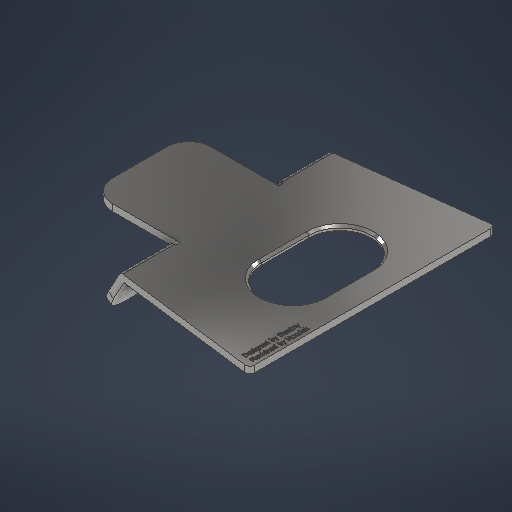
# Autodesk Inventor part: MK_5_rust_helma1
Saved by Autodesk Inventor 2025.3 (Build 293356000, 356)
## iProperties
Created: 2025-04-03
Part Number: MK_5_rust_helma1
Material: Ocel
Document SubType Name: Modeling
Designer: kolom_rupe2o
Density: 7.85 g/cm^3
Appearance: Ocel – leštěná
Author: kolom_rupe2o
Autodesk Inventor part; units mm, degrees
(part 1 of 2)
ref_plane "YZ Plane" through (0, 0, 0) normal (1, 0, 0) x (0, 1, 0)
ref_plane "XZ Plane" through (0, 0, 0) normal (0, 1, 0) x (-1, 0, 0)
ref_plane "XY Plane" through (0, 0, 0) normal (0, 0, 1) x (1, 0, 0)
sketch "Náčrt1" plane through (0, 0, 0) normal (0, 1, 0) x (-1, 0, 0)
  line L0 (0, 0) -> (0, -55)
  line L1 (0, -55) -> (32, -51)
  line L2 (32, -51) -> (32, -4)
  line L3 (32, -4) -> (0, 0)
  line L4 (12.5, -22.25) -> (12.5, -32.75) construction
  line L5 (5.5, -22.25) -> (5.5, -32.75)
  line L6 (19.5, -32.75) -> (19.5, -22.25)
  arc A0 (19.5, -22.25) -> (5.5, -22.25) centre (12.5, -22.25) ccw
  arc A1 (5.5, -32.75) -> (19.5, -32.75) centre (12.5, -32.75) ccw
  line L7 (32, -16.5) -> (52, -16.5)
  line L8 (52, -16.5) -> (52, -38.5)
  line L9 (52, -38.5) -> (32, -38.5)
  line L10 (32, -38.5) -> (32, -16.5)
  point P0 (32, -27.5)
  point P1 (0, -27.5)
  point P2 (12.5, -27.5)
  point P3 (52, -27.5)
  dimension "d0" = 47
  dimension "d1" = 55
  dimension "d2" = 32
  dimension "d3" = 12.5
  dimension "d4" = 7
  dimension "d5" = 10.5
  dimension "d6" = 22
  dimension "d7" = 20
  constraints: 24 end point, 4 midpoint, 4 parallel, 4 point on circle, 4 tangent, 3 horizontal alignment, 2 centre point, 2 vertical, 1 equal length, 1 horizontal, 1 perpendicular, 1 point on line
  measures "d0" distance of L1.end L2.end
  measures "d1" distance of L0.start L0.end
  measures "d2" distance between parallel lines of L0 L2
  measures "d3" distance between parallel lines of L2 L6
  measures "d4" radius of A1
  measures "d5" distance of L4.start L4.end
  measures "d6" distance of L7.end L8.end
  measures "d7" distance of L8.end L9.end
extrude "Vysunutí1" add sketch "Náčrt1" along normal blind 1.5
ref_plane "Pracovní rovina1" through (-52, 0, -27.5) normal (0, 0, 1) x (1, 0, 0)
ref_plane "Pracovní rovina2" through (-52, 0, -15.5) normal (0, 0, 1) x (1, 0, 0)
sketch "Náčrt3" plane through (-52, 0, -15.5) normal (0, 0, 1) x (1, 0, 0)
  line L0 (20, 0) -> (52, 0)
  line L1 (52, 0) -> (52, 1.5)
  line L2 (20, 1.5) -> (52, 1.5)
  line L3 (20, 0) -> (20, 1.5)
  line L4 (20, 0) -> (15, -8.6603)
  line L5 (15, -8.6603) -> (13.701, -7.9103)
  line L6 (13.701, -7.9103) -> (19.134, 1.5)
  line L7 (19.134, 1.5) -> (20, 1.5)
  line L8 (20, 0) -> (20, 1.5)
  line L9 (20, 0) -> (20, 1.5)
  dimension "d14" = 120
  dimension "d15" = 1.5
  dimension "d16" = 10
  constraints: 8 end point, 2 perpendicular, 1 collinear
  measures "d14" angle of L0 L4
  measures "d15" distance of L4.end L5.end
  measures "d16" distance of L0.start L4.end
extrude "Vysunutí2" add sketch "Náčrt3" along normal up to surface contours L4 L5 L6 L7 L3 surface through (-32, 0, -4) normal (-0.1240347, 0, 0.9922779)
sketch "Náčrt4" plane through (-32.866, 1.5, -15.5) normal (-0.8660254, 0.5, 0) x (0, 0, 1)
  line L0 (10.7126, -10.866) -> (11.3917, 0)
  line L1 (0, 0) -> (11.3917, 0)
  line L2 (0, 0) -> (0, -10.866)
  line L3 (0, -10.866) -> (10.7126, -10.866)
  point P0 (15.5, 15.134)
  point P1 (5.3563, -5.433)
  point P2 (0, -5.433)
  point P3 (5.3563, -10.866)
  constraints: 2 midpoint, 1 horizontal alignment, 1 vertical alignment
hole "Díra1" at (-35.5825, -3.2051, -10.1437) direction (0.8660254, -0.5, 0) diameter 3 end through all
mirror "Zrcadlit1" about plane through (-52, 0, -27.5) normal (0, 0, 1) of "Díra1", "Vysunutí2"
fillet "Zaoblení1" radius 1 2 edges at (-32.866, 1.5, -45.1959) (-32.866, 1.5, -9.8041)
fillet "Zaoblení2" radius 5 6 edges at (-37.6495, -8.2853, -4.7062) (-37.6495, -8.2853, -15.5) (-37.6495, -8.2853, -39.5) (-37.6495, -8.2853, -50.2938) (-52, 0.75, -16.5) (-52, 0.75, -38.5)
fillet "Zaoblení3" radius 1 2 edges at (0, 0.75, -55) (0, 0.75, 0)
chamfer "Zkosení1" distance 0.5 angle 45 8 edges at (-19.5, 1.5, -27.5) (-12.5, 1.5, -39.75) (-5.5, 1.5, -27.5) (-12.5, 1.5, -15.25) (-19.5, 0, -27.5) (-12.5, 0, -39.75) (-5.5, 0, -27.5) (-12.5, 0, -15.25)
sketch "Náčrt6" plane through (0, 1.5, 0) normal (0, 1, 0) x (1, 0, 0)
  arc A0 (-1.124, 0.1405) -> (0, 1.1328) centre (-1, 1.1328) ccw
  line L0 (0, 1.1328) -> (0, 53.8672)
  arc A1 (0, 53.8672) -> (-1.124, 54.8595) centre (-1, 53.8672) ccw
  line L1 (-1.124, 54.8595) -> (-32.2887, 50.9639)
  line L2 (-32.2887, 39.5) -> (-32.2887, 50.9639)
  line L3 (-32, 39.5) -> (-32.2887, 39.5)
  line L4 (-32, 39.5) -> (-32, 38.5)
  line L5 (-32, 38.5) -> (-47, 38.5)
  arc A2 (-47, 38.5) -> (-52, 33.5) centre (-47, 33.5) ccw
  line L6 (-52, 33.5) -> (-52, 21.5)
  arc A3 (-52, 21.5) -> (-47, 16.5) centre (-47, 21.5) ccw
  line L7 (-47, 16.5) -> (-32, 16.5)
  line L8 (-32, 16.5) -> (-32, 15.5)
  line L9 (-32, 15.5) -> (-32.2887, 15.5)
  line L10 (-32.2887, 4.0361) -> (-32.2887, 15.5)
  line L11 (-32.2887, 4.0361) -> (-1.124, 0.1405)
  line L12 (-20, 32.75) -> (-20, 22.25)
  arc A4 (-5, 32.75) -> (-20, 32.75) centre (-12.5, 32.75) ccw
  line L13 (-5, 22.25) -> (-5, 32.75)
  arc A5 (-20, 22.25) -> (-5, 22.25) centre (-12.5, 22.25) ccw
  line L14 (-3.5, 1.6328) -> (-3.5, 16.6328) construction
  line L15 (-3.5, 16.6328) -> (0, 16.6328) construction
  line L16 (0, 16.6328) -> (0, 1.6328) construction
  line L17 (0, 1.6328) -> (-3.5, 1.6328) construction
  spline S0 degree 2 poles (-2.9546, 2.5226) (-2.8177, 2.5226) (-2.5972, 2.4116) (-2.5357, 2.3184) knots 0 0 0 1 2 2 2
  spline S1 degree 2 poles (-2.5357, 2.3184) (-2.4878, 2.2422) (-2.4554, 2.0858) (-2.4554, 1.9642) knots 0 0 0 1 2 2 2
  line L18 (-2.4554, 1.9642) -> (-2.4554, 1.7341)
  line L19 (-2.4554, 1.7341) -> (-3.4554, 1.7341)
  line L20 (-3.4554, 1.7341) -> (-3.4554, 1.9618)
  spline S2 degree 2 poles (-3.4554, 1.9618) (-3.4554, 2.1028) (-3.4133, 2.2633) (-3.376, 2.32) knots 0 0 0 1 2 2 2
  spline S3 degree 2 poles (-3.376, 2.32) (-3.312, 2.4164) (-3.1005, 2.5226) (-2.9546, 2.5226) knots 0 0 0 1 2 2 2
  spline S4 degree 2 poles (-2.9562, 2.384) (-3.0713, 2.384) (-3.2342, 2.3078) (-3.2804, 2.2325) knots 0 0 0 1 2 2 2
  spline S5 degree 2 poles (-3.2804, 2.2325) (-3.312, 2.179) (-3.3404, 2.0582) (-3.3404, 1.9683) knots 0 0 0 1 2 2 2
  line L21 (-3.3404, 1.9683) -> (-3.3404, 1.867)
  line L22 (-3.3404, 1.867) -> (-2.5705, 1.867)
  line L23 (-2.5705, 1.867) -> (-2.5705, 1.9683)
  spline S6 degree 2 poles (-2.5705, 1.9683) (-2.5705, 2.0566) (-2.5989, 2.1903) (-2.637, 2.2446) knots 0 0 0 1 2 2 2
  spline S7 degree 2 poles (-2.637, 2.2446) (-2.684, 2.3143) (-2.8395, 2.384) (-2.9562, 2.384) knots 0 0 0 1 2 2 2
  spline S8 degree 2 poles (-2.4384, 2.9829) (-2.4384, 2.803) (-2.6402, 2.6052) (-2.8266, 2.6052) knots 0 0 0 1 2 2 2
  spline S9 degree 2 poles (-2.8266, 2.6052) (-3.0097, 2.6052) (-3.2269, 2.7973) (-3.2269, 2.9521) knots 0 0 0 1 2 2 2
  spline S10 degree 2 poles (-3.2269, 2.9521) (-3.2269, 3.0218) (-3.1864, 3.1295) (-3.1434, 3.1692) knots 0 0 0 1 2 2 2
  spline S11 degree 2 poles (-3.1434, 3.1692) (-3.1005, 3.2098) (-2.9765, 3.2527) (-2.8865, 3.2527) knots 0 0 0 1 2 2 2
  line L24 (-2.8865, 3.2527) -> (-2.8177, 3.2527)
  line L25 (-2.8177, 3.2527) -> (-2.8177, 2.7333)
  spline S12 degree 2 poles (-2.8177, 2.7333) (-2.6872, 2.7333) (-2.5486, 2.8645) (-2.5486, 2.9812) knots 0 0 0 1 2 2 2
  spline S13 degree 2 poles (-2.5486, 2.9812) (-2.5486, 3.0226) (-2.5673, 3.1028) (-2.5818, 3.1352) knots 0 0 0 1 2 2 2
  spline S14 degree 2 poles (-2.5818, 3.1352) (-2.5981, 3.1692) (-2.6264, 3.2163) (-2.6394, 3.2316) knots 0 0 0 1 2 2 2
  line L26 (-2.6394, 3.2316) -> (-2.6394, 3.2389)
  line L27 (-2.6394, 3.2389) -> (-2.5016, 3.2389)
  spline S15 degree 2 poles (-2.5016, 3.2389) (-2.4927, 3.2171) (-2.4668, 3.1506) (-2.4595, 3.1247) knots 0 0 0 1 2 2 2
  spline S16 degree 2 poles (-2.4595, 3.1247) (-2.4489, 3.0882) (-2.4384, 3.0282) (-2.4384, 2.9829) knots 0 0 0 1 2 2 2
  spline S17 degree 2 poles (-2.9141, 3.1295) (-2.9652, 3.1279) (-3.0397, 3.1069) (-3.0648, 3.0866) knots 0 0 0 1 2 2 2
  spline S18 degree 2 poles (-3.0648, 3.0866) (-3.0932, 3.0647) (-3.1232, 2.9958) (-3.1232, 2.9448) knots 0 0 0 1 2 2 2
  spline S19 degree 2 poles (-3.1232, 2.9448) (-3.1232, 2.8945) (-3.0932, 2.824) (-3.064, 2.7949) knots 0 0 0 1 2 2 2
  spline S20 degree 2 poles (-3.064, 2.7949) (-3.034, 2.7665) (-2.9619, 2.7373) (-2.9141, 2.7333) knots 0 0 0 1 2 2 2
  line L28 (-2.9141, 2.7333) -> (-2.9141, 3.1295)
  spline S21 degree 2 poles (-2.4376, 3.5833) (-2.4376, 3.508) (-2.4781, 3.3775) (-2.5008, 3.3346) knots 0 0 0 1 2 2 2
  line L29 (-2.5008, 3.3346) -> (-2.6426, 3.3346)
  line L30 (-2.6426, 3.3346) -> (-2.6426, 3.341)
  spline S22 degree 2 poles (-2.6426, 3.341) (-2.6297, 3.3573) (-2.5989, 3.401) (-2.5818, 3.4375) knots 0 0 0 1 2 2 2
  spline S23 degree 2 poles (-2.5818, 3.4375) (-2.5665, 3.4691) (-2.5438, 3.5469) (-2.5438, 3.5882) knots 0 0 0 1 2 2 2
  spline S24 degree 2 poles (-2.5438, 3.5882) (-2.5438, 3.6182) (-2.5575, 3.6871) (-2.5689, 3.7033) knots 0 0 0 1 2 2 2
  spline S25 degree 2 poles (-2.5689, 3.7033) (-2.5843, 3.7268) (-2.6191, 3.7479) (-2.6548, 3.7479) knots 0 0 0 1 2 2 2
  spline S26 degree 2 poles (-2.6548, 3.7479) (-2.6994, 3.7479) (-2.7455, 3.6992) (-2.7609, 3.6368) knots 0 0 0 1 2 2 2
  spline S27 degree 2 poles (-2.7609, 3.6368) (-2.7666, 3.6125) (-2.7828, 3.5347) (-2.7917, 3.5015) knots 0 0 0 1 2 2 2
  spline S28 degree 2 poles (-2.7917, 3.5015) (-2.8169, 3.4156) (-2.9206, 3.3378) (-2.9943, 3.3378) knots 0 0 0 1 2 2 2
  spline S29 degree 2 poles (-2.9943, 3.3378) (-3.0964, 3.3378) (-3.2237, 3.491) (-3.2237, 3.6174) knots 0 0 0 1 2 2 2
  spline S30 degree 2 poles (-3.2237, 3.6174) (-3.2237, 3.6798) (-3.1929, 3.8062) (-3.1694, 3.8492) knots 0 0 0 1 2 2 2
  line L31 (-3.1694, 3.8492) -> (-3.034, 3.8492)
  line L32 (-3.034, 3.8492) -> (-3.034, 3.8427)
  spline S31 degree 2 poles (-3.034, 3.8427) (-3.0729, 3.794) (-3.1175, 3.6757) (-3.1175, 3.615) knots 0 0 0 1 2 2 2
  spline S32 degree 2 poles (-3.1175, 3.615) (-3.1175, 3.5526) (-3.0648, 3.4667) (-3.0122, 3.4667) knots 0 0 0 1 2 2 2
  spline S33 degree 2 poles (-3.0122, 3.4667) (-2.9643, 3.4667) (-2.9182, 3.5177) (-2.9036, 3.5744) knots 0 0 0 1 2 2 2
  spline S34 degree 2 poles (-2.9036, 3.5744) (-2.8963, 3.602) (-2.8817, 3.6717) (-2.8728, 3.7098) knots 0 0 0 1 2 2 2
  spline S35 degree 2 poles (-2.8728, 3.7098) (-2.8517, 3.7924) (-2.7553, 3.8767) (-2.6718, 3.8767) knots 0 0 0 1 2 2 2
  spline S36 degree 2 poles (-2.6718, 3.8767) (-2.6232, 3.8767) (-2.5373, 3.8386) (-2.5057, 3.8013) knots 0 0 0 1 2 2 2
  spline S37 degree 2 poles (-2.5057, 3.8013) (-2.4724, 3.7616) (-2.4376, 3.6603) (-2.4376, 3.5833) knots 0 0 0 1 2 2 2
  line L33 (-2.4554, 4.1231) -> (-2.4554, 3.9966)
  line L34 (-2.4554, 3.9966) -> (-3.2058, 3.9966)
  line L35 (-3.2058, 3.9966) -> (-3.2058, 4.1231)
  line L36 (-3.2058, 4.1231) -> (-2.4554, 4.1231)
  line L37 (-3.3306, 4.132) -> (-3.3306, 3.9885)
  line L38 (-3.3306, 3.9885) -> (-3.4619, 3.9885)
  line L39 (-3.4619, 3.9885) -> (-3.4619, 4.132)
  line L40 (-3.4619, 4.132) -> (-3.3306, 4.132)
  spline S38 degree 2 poles (-2.3355, 4.3354) (-2.3298, 4.3483) (-2.312, 4.3978) (-2.3047, 4.4294) knots 0 0 0 1 2 2 2
  spline S39 degree 2 poles (-2.3047, 4.4294) (-2.2958, 4.4642) (-2.2853, 4.5234) (-2.2853, 4.5582) knots 0 0 0 1 2 2 2
  spline S40 degree 2 poles (-2.2853, 4.5582) (-2.2853, 4.6166) (-2.316, 4.6976) (-2.3436, 4.7203) knots 0 0 0 1 2 2 2
  spline S41 degree 2 poles (-2.3436, 4.7203) (-2.3712, 4.7422) (-2.4433, 4.7592) (-2.4895, 4.7592) knots 0 0 0 1 2 2 2
  line L41 (-2.4895, 4.7592) -> (-2.5551, 4.7592)
  spline S42 degree 2 poles (-2.5551, 4.7592) (-2.5105, 4.7081) (-2.4684, 4.6101) (-2.4684, 4.5363) knots 0 0 0 1 2 2 2
  spline S43 degree 2 poles (-2.4684, 4.5363) (-2.4684, 4.4083) (-2.6588, 4.2568) (-2.8379, 4.2568) knots 0 0 0 1 2 2 2
  spline S44 degree 2 poles (-2.8379, 4.2568) (-2.9311, 4.2568) (-3.0754, 4.3094) (-3.1264, 4.3532) knots 0 0 0 1 2 2 2
  spline S45 degree 2 poles (-3.1264, 4.3532) (-3.1742, 4.3953) (-3.2269, 4.5112) (-3.2269, 4.5728) knots 0 0 0 1 2 2 2
  spline S46 degree 2 poles (-3.2269, 4.5728) (-3.2269, 4.6312) (-3.1994, 4.7163) (-3.1742, 4.7592) knots 0 0 0 1 2 2 2
  line L42 (-3.1742, 4.7592) -> (-3.2058, 4.7665)
  line L43 (-3.2058, 4.7665) -> (-3.2058, 4.8856)
  line L44 (-3.2058, 4.8856) -> (-2.5413, 4.8856)
  spline S47 degree 2 poles (-2.5413, 4.8856) (-2.3501, 4.8856) (-2.1718, 4.7195) (-2.1718, 4.5485) knots 0 0 0 1 2 2 2
  spline S48 degree 2 poles (-2.1718, 4.5485) (-2.1718, 4.4934) (-2.1896, 4.3783) (-2.2042, 4.3289) knots 0 0 0 1 2 2 2
  line L45 (-2.2042, 4.3289) -> (-2.3355, 4.3289)
  line L46 (-2.3355, 4.3289) -> (-2.3355, 4.3354)
  line L47 (-2.6588, 4.7592) -> (-3.0713, 4.7592)
  spline S49 degree 2 poles (-3.0713, 4.7592) (-3.094, 4.7122) (-3.1135, 4.6328) (-3.1135, 4.5931) knots 0 0 0 1 2 2 2
  spline S50 degree 2 poles (-3.1135, 4.5931) (-3.1135, 4.4975) (-2.9724, 4.3872) (-2.8404, 4.3872) knots 0 0 0 1 2 2 2
  spline S51 degree 2 poles (-2.8404, 4.3872) (-2.7156, 4.3872) (-2.5851, 4.4707) (-2.5851, 4.5647) knots 0 0 0 1 2 2 2
  spline S52 degree 2 poles (-2.5851, 4.5647) (-2.5851, 4.6141) (-2.624, 4.7179) (-2.6588, 4.7592) knots 0 0 0 1 2 2 2
  line L48 (-2.4554, 5.6579) -> (-2.4554, 5.5315)
  line L49 (-2.4554, 5.5315) -> (-2.8833, 5.5315)
  spline S53 degree 2 poles (-2.8833, 5.5315) (-2.9352, 5.5315) (-3.0243, 5.5218) (-3.0511, 5.5072) knots 0 0 0 1 2 2 2
  spline S54 degree 2 poles (-3.0511, 5.5072) (-3.0794, 5.4918) (-3.107, 5.4367) (-3.107, 5.3897) knots 0 0 0 1 2 2 2
  spline S55 degree 2 poles (-3.107, 5.3897) (-3.107, 5.3427) (-3.0567, 5.243) (-3.0162, 5.1952) knots 0 0 0 1 2 2 2
  line L50 (-3.0162, 5.1952) -> (-2.4554, 5.1952)
  line L51 (-2.4554, 5.1952) -> (-2.4554, 5.0688)
  line L52 (-2.4554, 5.0688) -> (-3.2058, 5.0688)
  line L53 (-3.2058, 5.0688) -> (-3.2058, 5.1952)
  line L54 (-3.2058, 5.1952) -> (-3.1224, 5.1952)
  spline S56 degree 2 poles (-3.1224, 5.1952) (-3.1734, 5.2519) (-3.2269, 5.3613) (-3.2269, 5.4229) knots 0 0 0 1 2 2 2
  spline S57 degree 2 poles (-3.2269, 5.4229) (-3.2269, 5.5331) (-3.081, 5.6579) (-2.9425, 5.6579) knots 0 0 0 1 2 2 2
  line L55 (-2.9425, 5.6579) -> (-2.4554, 5.6579)
  spline S58 degree 2 poles (-2.4384, 6.1611) (-2.4384, 5.9812) (-2.6402, 5.7835) (-2.8266, 5.7835) knots 0 0 0 1 2 2 2
  spline S59 degree 2 poles (-2.8266, 5.7835) (-3.0097, 5.7835) (-3.2269, 5.9756) (-3.2269, 6.1304) knots 0 0 0 1 2 2 2
  spline S60 degree 2 poles (-3.2269, 6.1304) (-3.2269, 6.2) (-3.1864, 6.3078) (-3.1434, 6.3475) knots 0 0 0 1 2 2 2
  spline S61 degree 2 poles (-3.1434, 6.3475) (-3.1005, 6.388) (-2.9765, 6.431) (-2.8865, 6.431) knots 0 0 0 1 2 2 2
  line L56 (-2.8865, 6.431) -> (-2.8177, 6.431)
  line L57 (-2.8177, 6.431) -> (-2.8177, 5.9116)
  spline S62 degree 2 poles (-2.8177, 5.9116) (-2.6872, 5.9116) (-2.5486, 6.0428) (-2.5486, 6.1595) knots 0 0 0 1 2 2 2
  spline S63 degree 2 poles (-2.5486, 6.1595) (-2.5486, 6.2009) (-2.5673, 6.2811) (-2.5818, 6.3135) knots 0 0 0 1 2 2 2
  spline S64 degree 2 poles (-2.5818, 6.3135) (-2.5981, 6.3475) (-2.6264, 6.3945) (-2.6394, 6.4099) knots 0 0 0 1 2 2 2
  line L58 (-2.6394, 6.4099) -> (-2.6394, 6.4172)
  line L59 (-2.6394, 6.4172) -> (-2.5016, 6.4172)
  spline S65 degree 2 poles (-2.5016, 6.4172) (-2.4927, 6.3953) (-2.4668, 6.3289) (-2.4595, 6.303) knots 0 0 0 1 2 2 2
  spline S66 degree 2 poles (-2.4595, 6.303) (-2.4489, 6.2665) (-2.4384, 6.2065) (-2.4384, 6.1611) knots 0 0 0 1 2 2 2
  spline S67 degree 2 poles (-2.9141, 6.3078) (-2.9652, 6.3062) (-3.0397, 6.2851) (-3.0648, 6.2649) knots 0 0 0 1 2 2 2
  spline S68 degree 2 poles (-3.0648, 6.2649) (-3.0932, 6.243) (-3.1232, 6.1741) (-3.1232, 6.1231) knots 0 0 0 1 2 2 2
  spline S69 degree 2 poles (-3.1232, 6.1231) (-3.1232, 6.0728) (-3.0932, 6.0023) (-3.064, 5.9731) knots 0 0 0 1 2 2 2
  spline S70 degree 2 poles (-3.064, 5.9731) (-3.034, 5.9448) (-2.9619, 5.9156) (-2.9141, 5.9116) knots 0 0 0 1 2 2 2
  line L60 (-2.9141, 5.9116) -> (-2.9141, 6.3078)
  line L61 (-2.4554, 7.136) -> (-2.4554, 7.0096)
  line L62 (-2.4554, 7.0096) -> (-2.5316, 7.0096)
  spline S71 degree 2 poles (-2.5316, 7.0096) (-2.5073, 6.9804) (-2.4749, 6.9375) (-2.4611, 6.9083) knots 0 0 0 1 2 2 2
  spline S72 degree 2 poles (-2.4611, 6.9083) (-2.4481, 6.8816) (-2.4344, 6.824) (-2.4344, 6.7859) knots 0 0 0 1 2 2 2
  spline S73 degree 2 poles (-2.4344, 6.7859) (-2.4344, 6.7244) (-2.4854, 6.6206) (-2.5348, 6.5842) knots 0 0 0 1 2 2 2
  spline S74 degree 2 poles (-2.5348, 6.5842) (-2.5843, 6.5477) (-2.7301, 6.5072) (-2.825, 6.5072) knots 0 0 0 1 2 2 2
  spline S75 degree 2 poles (-2.825, 6.5072) (-2.9238, 6.5072) (-3.0681, 6.5582) (-3.1224, 6.6028) knots 0 0 0 1 2 2 2
  spline S76 degree 2 poles (-3.1224, 6.6028) (-3.171, 6.6441) (-3.2269, 6.76) (-3.2269, 6.824) knots 0 0 0 1 2 2 2
  spline S77 degree 2 poles (-3.2269, 6.824) (-3.2269, 6.8799) (-3.2018, 6.9634) (-3.1759, 7.0096) knots 0 0 0 1 2 2 2
  line L63 (-3.1759, 7.0096) -> (-3.5, 7.0096)
  line L64 (-3.5, 7.0096) -> (-3.5, 7.136)
  line L65 (-3.5, 7.136) -> (-2.4554, 7.136)
  line L66 (-2.6378, 7.0096) -> (-3.0713, 7.0096)
  spline S78 degree 2 poles (-3.0713, 7.0096) (-3.094, 6.9626) (-3.111, 6.888) (-3.111, 6.8451) knots 0 0 0 1 2 2 2
  spline S79 degree 2 poles (-3.111, 6.8451) (-3.111, 6.7479) (-2.9652, 6.6376) (-2.8274, 6.6376) knots 0 0 0 1 2 2 2
  spline S80 degree 2 poles (-2.8274, 6.6376) (-2.6945, 6.6376) (-2.5543, 6.7219) (-2.5543, 6.8151) knots 0 0 0 1 2 2 2
  spline S81 degree 2 poles (-2.5543, 6.8151) (-2.5543, 6.8645) (-2.5997, 6.965) (-2.6378, 7.0096) knots 0 0 0 1 2 2 2
  spline S82 degree 2 poles (-2.8428, 8.3775) (-2.6588, 8.3775) (-2.4344, 8.1992) (-2.4344, 8.0647) knots 0 0 0 1 2 2 2
  spline S83 degree 2 poles (-2.4344, 8.0647) (-2.4344, 8.0039) (-2.4643, 7.9172) (-2.4903, 7.8751) knots 0 0 0 1 2 2 2
  line L67 (-2.4903, 7.8751) -> (-2.4554, 7.867)
  line L68 (-2.4554, 7.867) -> (-2.4554, 7.7487)
  line L69 (-2.4554, 7.7487) -> (-3.5, 7.7487)
  line L70 (-3.5, 7.7487) -> (-3.5, 7.8751)
  line L71 (-3.5, 7.8751) -> (-3.1272, 7.8751)
  spline S84 degree 2 poles (-3.1272, 7.8751) (-3.1702, 7.9229) (-3.2269, 8.0339) (-3.2269, 8.1044) knots 0 0 0 1 2 2 2
  spline S85 degree 2 poles (-3.2269, 8.1044) (-3.2269, 8.2316) (-3.0235, 8.3775) (-2.8428, 8.3775) knots 0 0 0 1 2 2 2
  spline S86 degree 2 poles (-2.8331, 8.247) (-2.9676, 8.247) (-3.107, 8.1652) (-3.107, 8.0744) knots 0 0 0 1 2 2 2
  spline S87 degree 2 poles (-3.107, 8.0744) (-3.107, 8.0234) (-3.0583, 7.918) (-3.0211, 7.8751) knots 0 0 0 1 2 2 2
  line L72 (-3.0211, 7.8751) -> (-2.5908, 7.8751)
  spline S88 degree 2 poles (-2.5908, 7.8751) (-2.5673, 7.9229) (-2.5478, 7.9966) (-2.5478, 8.0404) knots 0 0 0 1 2 2 2
  spline S89 degree 2 poles (-2.5478, 8.0404) (-2.5478, 8.1368) (-2.6848, 8.247) (-2.8331, 8.247) knots 0 0 0 1 2 2 2
  line L73 (-3.2058, 9.0979) -> (-2.1791, 8.6944)
  line L74 (-2.1791, 8.6944) -> (-2.1791, 8.559)
  line L75 (-2.1791, 8.559) -> (-2.4919, 8.6936)
  line L76 (-2.4919, 8.6936) -> (-3.2058, 8.4213)
  line L77 (-3.2058, 8.4213) -> (-3.2058, 8.5574)
  line L78 (-3.2058, 8.5574) -> (-2.6499, 8.7624)
  line L79 (-2.6499, 8.7624) -> (-3.2058, 8.9667)
  line L80 (-3.2058, 8.9667) -> (-3.2058, 9.0979)
  spline S90 degree 2 poles (-2.4376, 9.9116) (-2.4376, 9.803) (-2.483, 9.6506) (-2.5154, 9.5833) knots 0 0 0 1 2 2 2
  line L81 (-2.5154, 9.5833) -> (-2.6823, 9.5833)
  line L82 (-2.6823, 9.5833) -> (-2.6823, 9.5931)
  spline S91 degree 2 poles (-2.6823, 9.5931) (-2.6207, 9.6587) (-2.5527, 9.8248) (-2.5527, 9.9018) knots 0 0 0 1 2 2 2
  spline S92 degree 2 poles (-2.5527, 9.9018) (-2.5527, 10.012) (-2.6442, 10.1247) (-2.7196, 10.1247) knots 0 0 0 1 2 2 2
  spline S93 degree 2 poles (-2.7196, 10.1247) (-2.7796, 10.1247) (-2.8541, 10.0655) (-2.8728, 10.0015) knots 0 0 0 1 2 2 2
  spline S94 degree 2 poles (-2.8728, 10.0015) (-2.8857, 9.9553) (-2.9036, 9.8783) (-2.9182, 9.8208) knots 0 0 0 1 2 2 2
  spline S95 degree 2 poles (-2.9182, 9.8208) (-2.9319, 9.7689) (-2.9733, 9.6871) (-3.0065, 9.6555) knots 0 0 0 1 2 2 2
  spline S96 degree 2 poles (-3.0065, 9.6555) (-3.0397, 9.6247) (-3.1288, 9.5906) (-3.1872, 9.5906) knots 0 0 0 1 2 2 2
  spline S97 degree 2 poles (-3.1872, 9.5906) (-3.3088, 9.5906) (-3.4733, 9.7803) (-3.4733, 9.9269) knots 0 0 0 1 2 2 2
  spline S98 degree 2 poles (-3.4733, 9.9269) (-3.4733, 10.0112) (-3.44, 10.1603) (-3.4084, 10.2244) knots 0 0 0 1 2 2 2
  line L83 (-3.4084, 10.2244) -> (-3.2496, 10.2244)
  line L84 (-3.2496, 10.2244) -> (-3.2496, 10.2146)
  spline S99 degree 2 poles (-3.2496, 10.2146) (-3.2934, 10.1668) (-3.3582, 10.0177) (-3.3582, 9.9359) knots 0 0 0 1 2 2 2
  spline S100 degree 2 poles (-3.3582, 9.9359) (-3.3582, 9.8435) (-3.2715, 9.7292) (-3.201, 9.7292) knots 0 0 0 1 2 2 2
  spline S101 degree 2 poles (-3.201, 9.7292) (-3.1378, 9.7292) (-3.0624, 9.7965) (-3.0454, 9.8597) knots 0 0 0 1 2 2 2
  spline S102 degree 2 poles (-3.0454, 9.8597) (-3.034, 9.9018) (-3.0049, 10.0242) (-2.9927, 10.0647) knots 0 0 0 1 2 2 2
  spline S103 degree 2 poles (-2.9927, 10.0647) (-2.9611, 10.1676) (-2.8339, 10.2633) (-2.7407, 10.2633) knots 0 0 0 1 2 2 2
  spline S104 degree 2 poles (-2.7407, 10.2633) (-2.6815, 10.2633) (-2.5681, 10.2154) (-2.5284, 10.1725) knots 0 0 0 1 2 2 2
  spline S105 degree 2 poles (-2.5284, 10.1725) (-2.4846, 10.1247) (-2.4376, 10.0031) (-2.4376, 9.9116) knots 0 0 0 1 2 2 2
  spline S106 degree 2 poles (-2.4408, 10.6158) (-2.4408, 10.5128) (-2.5583, 10.397) (-2.6856, 10.397) knots 0 0 0 1 2 2 2
  line L85 (-2.6856, 10.397) -> (-3.1013, 10.397)
  line L86 (-3.1013, 10.397) -> (-3.1013, 10.3119)
  line L87 (-3.1013, 10.3119) -> (-3.2058, 10.3119)
  line L88 (-3.2058, 10.3119) -> (-3.2058, 10.397)
  line L89 (-3.2058, 10.397) -> (-3.4214, 10.397)
  line L90 (-3.4214, 10.397) -> (-3.4214, 10.5234)
  line L91 (-3.4214, 10.5234) -> (-3.2058, 10.5234)
  line L92 (-3.2058, 10.5234) -> (-3.2058, 10.756)
  line L93 (-3.2058, 10.756) -> (-3.1013, 10.756)
  line L94 (-3.1013, 10.756) -> (-3.1013, 10.5234)
  line L95 (-3.1013, 10.5234) -> (-2.7439, 10.5234)
  spline S107 degree 2 poles (-2.7439, 10.5234) (-2.6872, 10.5234) (-2.6248, 10.5274) (-2.5981, 10.5412) knots 0 0 0 1 2 2 2
  spline S108 degree 2 poles (-2.5981, 10.5412) (-2.5746, 10.5526) (-2.5511, 10.6036) (-2.5511, 10.6474) knots 0 0 0 1 2 2 2
  spline S109 degree 2 poles (-2.5511, 10.6474) (-2.5511, 10.6782) (-2.5697, 10.7357) (-2.5754, 10.7487) knots 0 0 0 1 2 2 2
  line L96 (-2.5754, 10.7487) -> (-2.5754, 10.756)
  line L97 (-2.5754, 10.756) -> (-2.4619, 10.756)
  spline S110 degree 2 poles (-2.4619, 10.756) (-2.4522, 10.7203) (-2.4408, 10.6474) (-2.4408, 10.6158) knots 0 0 0 1 2 2 2
  spline S111 degree 2 poles (-2.5348, 11.2673) (-2.5235, 11.2519) (-2.483, 11.2) (-2.4708, 11.1757) knots 0 0 0 1 2 2 2
  spline S112 degree 2 poles (-2.4708, 11.1757) (-2.453, 11.1425) (-2.4344, 11.0801) (-2.4344, 11.0234) knots 0 0 0 1 2 2 2
  spline S113 degree 2 poles (-2.4344, 11.0234) (-2.4344, 10.9772) (-2.4692, 10.8937) (-2.5008, 10.8621) knots 0 0 0 1 2 2 2
  spline S114 degree 2 poles (-2.5008, 10.8621) (-2.5316, 10.8321) (-2.6224, 10.7957) (-2.6726, 10.7957) knots 0 0 0 1 2 2 2
  spline S115 degree 2 poles (-2.6726, 10.7957) (-2.7504, 10.7957) (-2.8606, 10.8613) (-2.8922, 10.9326) knots 0 0 0 1 2 2 2
  spline S116 degree 2 poles (-2.8922, 10.9326) (-2.9214, 10.9958) (-2.9433, 11.1676) (-2.9489, 11.2673) knots 0 0 0 1 2 2 2
  line L98 (-2.9489, 11.2673) -> (-2.9733, 11.2673)
  spline S117 degree 2 poles (-2.9733, 11.2673) (-3.017, 11.2673) (-3.0713, 11.2406) (-3.0867, 11.2163) knots 0 0 0 1 2 2 2
  spline S118 degree 2 poles (-3.0867, 11.2163) (-3.1021, 11.1919) (-3.1118, 11.1222) (-3.1118, 11.085) knots 0 0 0 1 2 2 2
  spline S119 degree 2 poles (-3.1118, 11.085) (-3.1118, 11.0412) (-3.0859, 10.9229) (-3.0608, 10.8637) knots 0 0 0 1 2 2 2
  line L99 (-3.0608, 10.8637) -> (-3.0608, 10.8564)
  line L100 (-3.0608, 10.8564) -> (-3.1896, 10.8564)
  spline S120 degree 2 poles (-3.1896, 10.8564) (-3.1994, 10.8913) (-3.2237, 11.0218) (-3.2237, 11.0858) knots 0 0 0 1 2 2 2
  spline S121 degree 2 poles (-3.2237, 11.0858) (-3.2237, 11.1636) (-3.1994, 11.2697) (-3.1677, 11.3119) knots 0 0 0 1 2 2 2
  spline S122 degree 2 poles (-3.1677, 11.3119) (-3.137, 11.3532) (-3.0389, 11.3937) (-2.9684, 11.3937) knots 0 0 0 1 2 2 2
  line L101 (-2.9684, 11.3937) -> (-2.4554, 11.3937)
  line L102 (-2.4554, 11.3937) -> (-2.4554, 11.2673)
  line L103 (-2.4554, 11.2673) -> (-2.5348, 11.2673)
  line L104 (-2.6402, 11.2673) -> (-2.8485, 11.2673)
  spline S123 degree 2 poles (-2.8485, 11.2673) (-2.8444, 11.2219) (-2.8306, 11.085) (-2.8177, 11.042) knots 0 0 0 1 2 2 2
  spline S124 degree 2 poles (-2.8177, 11.042) (-2.8023, 10.9918) (-2.7382, 10.9261) (-2.6815, 10.9261) knots 0 0 0 1 2 2 2
  spline S125 degree 2 poles (-2.6815, 10.9261) (-2.6167, 10.9261) (-2.5511, 10.9991) (-2.5511, 11.0688) knots 0 0 0 1 2 2 2
  spline S126 degree 2 poles (-2.5511, 11.0688) (-2.5511, 11.1279) (-2.6021, 11.2252) (-2.6402, 11.2673) knots 0 0 0 1 2 2 2
  spline S127 degree 2 poles (-2.4376, 11.7738) (-2.4376, 11.6984) (-2.4781, 11.568) (-2.5008, 11.525) knots 0 0 0 1 2 2 2
  line L105 (-2.5008, 11.525) -> (-2.6426, 11.525)
  line L106 (-2.6426, 11.525) -> (-2.6426, 11.5315)
  spline S128 degree 2 poles (-2.6426, 11.5315) (-2.6297, 11.5477) (-2.5989, 11.5915) (-2.5818, 11.6279) knots 0 0 0 1 2 2 2
  spline S129 degree 2 poles (-2.5818, 11.6279) (-2.5665, 11.6595) (-2.5438, 11.7373) (-2.5438, 11.7786) knots 0 0 0 1 2 2 2
  spline S130 degree 2 poles (-2.5438, 11.7786) (-2.5438, 11.8086) (-2.5575, 11.8775) (-2.5689, 11.8937) knots 0 0 0 1 2 2 2
  spline S131 degree 2 poles (-2.5689, 11.8937) (-2.5843, 11.9172) (-2.6191, 11.9383) (-2.6548, 11.9383) knots 0 0 0 1 2 2 2
  spline S132 degree 2 poles (-2.6548, 11.9383) (-2.6994, 11.9383) (-2.7455, 11.8897) (-2.7609, 11.8273) knots 0 0 0 1 2 2 2
  spline S133 degree 2 poles (-2.7609, 11.8273) (-2.7666, 11.803) (-2.7828, 11.7252) (-2.7917, 11.6919) knots 0 0 0 1 2 2 2
  spline S134 degree 2 poles (-2.7917, 11.6919) (-2.8169, 11.606) (-2.9206, 11.5282) (-2.9943, 11.5282) knots 0 0 0 1 2 2 2
  spline S135 degree 2 poles (-2.9943, 11.5282) (-3.0964, 11.5282) (-3.2237, 11.6814) (-3.2237, 11.8078) knots 0 0 0 1 2 2 2
  spline S136 degree 2 poles (-3.2237, 11.8078) (-3.2237, 11.8702) (-3.1929, 11.9966) (-3.1694, 12.0396) knots 0 0 0 1 2 2 2
  line L107 (-3.1694, 12.0396) -> (-3.034, 12.0396)
  line L108 (-3.034, 12.0396) -> (-3.034, 12.0331)
  spline S137 degree 2 poles (-3.034, 12.0331) (-3.0729, 11.9845) (-3.1175, 11.8662) (-3.1175, 11.8054) knots 0 0 0 1 2 2 2
  spline S138 degree 2 poles (-3.1175, 11.8054) (-3.1175, 11.743) (-3.0648, 11.6571) (-3.0122, 11.6571) knots 0 0 0 1 2 2 2
  spline S139 degree 2 poles (-3.0122, 11.6571) (-2.9643, 11.6571) (-2.9182, 11.7081) (-2.9036, 11.7649) knots 0 0 0 1 2 2 2
  spline S140 degree 2 poles (-2.9036, 11.7649) (-2.8963, 11.7924) (-2.8817, 11.8621) (-2.8728, 11.9002) knots 0 0 0 1 2 2 2
  spline S141 degree 2 poles (-2.8728, 11.9002) (-2.8517, 11.9829) (-2.7553, 12.0671) (-2.6718, 12.0671) knots 0 0 0 1 2 2 2
  spline S142 degree 2 poles (-2.6718, 12.0671) (-2.6232, 12.0671) (-2.5373, 12.0291) (-2.5057, 11.9918) knots 0 0 0 1 2 2 2
  spline S143 degree 2 poles (-2.5057, 11.9918) (-2.4724, 11.9521) (-2.4376, 11.8508) (-2.4376, 11.7738) knots 0 0 0 1 2 2 2
  spline S144 degree 2 poles (-2.4408, 12.4116) (-2.4408, 12.3086) (-2.5583, 12.1927) (-2.6856, 12.1927) knots 0 0 0 1 2 2 2
  line L109 (-2.6856, 12.1927) -> (-3.1013, 12.1927)
  line L110 (-3.1013, 12.1927) -> (-3.1013, 12.1077)
  line L111 (-3.1013, 12.1077) -> (-3.2058, 12.1077)
  line L112 (-3.2058, 12.1077) -> (-3.2058, 12.1927)
  line L113 (-3.2058, 12.1927) -> (-3.4214, 12.1927)
  line L114 (-3.4214, 12.1927) -> (-3.4214, 12.3192)
  line L115 (-3.4214, 12.3192) -> (-3.2058, 12.3192)
  line L116 (-3.2058, 12.3192) -> (-3.2058, 12.5517)
  line L117 (-3.2058, 12.5517) -> (-3.1013, 12.5517)
  line L118 (-3.1013, 12.5517) -> (-3.1013, 12.3192)
  line L119 (-3.1013, 12.3192) -> (-2.7439, 12.3192)
  spline S145 degree 2 poles (-2.7439, 12.3192) (-2.6872, 12.3192) (-2.6248, 12.3232) (-2.5981, 12.337) knots 0 0 0 1 2 2 2
  spline S146 degree 2 poles (-2.5981, 12.337) (-2.5746, 12.3483) (-2.5511, 12.3994) (-2.5511, 12.4432) knots 0 0 0 1 2 2 2
  spline S147 degree 2 poles (-2.5511, 12.4432) (-2.5511, 12.4739) (-2.5697, 12.5315) (-2.5754, 12.5445) knots 0 0 0 1 2 2 2
  line L120 (-2.5754, 12.5445) -> (-2.5754, 12.5517)
  line L121 (-2.5754, 12.5517) -> (-2.4619, 12.5517)
  spline S148 degree 2 poles (-2.4619, 12.5517) (-2.4522, 12.5161) (-2.4408, 12.4432) (-2.4408, 12.4116) knots 0 0 0 1 2 2 2
  line L122 (-2.4554, 13.2341) -> (-2.4554, 13.1077)
  line L123 (-2.4554, 13.1077) -> (-2.8833, 13.1077)
  spline S149 degree 2 poles (-2.8833, 13.1077) (-2.9352, 13.1077) (-3.0243, 13.0979) (-3.0511, 13.0833) knots 0 0 0 1 2 2 2
  spline S150 degree 2 poles (-3.0511, 13.0833) (-3.0794, 13.068) (-3.107, 13.0128) (-3.107, 12.9658) knots 0 0 0 1 2 2 2
  spline S151 degree 2 poles (-3.107, 12.9658) (-3.107, 12.9188) (-3.0567, 12.8192) (-3.0162, 12.7714) knots 0 0 0 1 2 2 2
  line L124 (-3.0162, 12.7714) -> (-2.4554, 12.7714)
  line L125 (-2.4554, 12.7714) -> (-2.4554, 12.6449)
  line L126 (-2.4554, 12.6449) -> (-3.2058, 12.6449)
  line L127 (-3.2058, 12.6449) -> (-3.2058, 12.7714)
  line L128 (-3.2058, 12.7714) -> (-3.1224, 12.7714)
  spline S152 degree 2 poles (-3.1224, 12.7714) (-3.1734, 12.8281) (-3.2269, 12.9375) (-3.2269, 12.9991) knots 0 0 0 1 2 2 2
  spline S153 degree 2 poles (-3.2269, 12.9991) (-3.2269, 13.1093) (-3.081, 13.2341) (-2.9425, 13.2341) knots 0 0 0 1 2 2 2
  line L129 (-2.9425, 13.2341) -> (-2.4554, 13.2341)
  line L130 (-3.2058, 14.0007) -> (-2.1791, 13.5971)
  line L131 (-2.1791, 13.5971) -> (-2.1791, 13.4618)
  line L132 (-2.1791, 13.4618) -> (-2.4919, 13.5963)
  line L133 (-2.4919, 13.5963) -> (-3.2058, 13.324)
  line L134 (-3.2058, 13.324) -> (-3.2058, 13.4602)
  line L135 (-3.2058, 13.4602) -> (-2.6499, 13.6652)
  line L136 (-2.6499, 13.6652) -> (-3.2058, 13.8694)
  line L137 (-3.2058, 13.8694) -> (-3.2058, 14.0007)
  line L138 (-0.809, 2.5915) -> (-0.809, 2.4586)
  line L139 (-0.809, 2.4586) -> (-1.6704, 2.4586)
  line L140 (-1.6704, 2.4586) -> (-1.0845, 2.1976)
  line L141 (-1.0845, 2.1976) -> (-1.0845, 2.1166)
  line L142 (-1.0845, 2.1166) -> (-1.6704, 1.8581)
  line L143 (-1.6704, 1.8581) -> (-0.809, 1.8581)
  line L144 (-0.809, 1.8581) -> (-0.809, 1.7341)
  line L145 (-0.809, 1.7341) -> (-1.809, 1.7341)
  line L146 (-1.809, 1.7341) -> (-1.809, 1.9156)
  line L147 (-1.809, 1.9156) -> (-1.2522, 2.1652)
  line L148 (-1.2522, 2.1652) -> (-1.809, 2.4067)
  line L149 (-1.809, 2.4067) -> (-1.809, 2.5915)
  line L150 (-1.809, 2.5915) -> (-0.809, 2.5915)
  spline S154 degree 2 poles (-0.8884, 3.2025) (-0.877, 3.1871) (-0.8365, 3.1352) (-0.8244, 3.1109) knots 0 0 0 1 2 2 2
  spline S155 degree 2 poles (-0.8244, 3.1109) (-0.8065, 3.0777) (-0.7879, 3.0153) (-0.7879, 2.9586) knots 0 0 0 1 2 2 2
  spline S156 degree 2 poles (-0.7879, 2.9586) (-0.7879, 2.9124) (-0.8227, 2.8289) (-0.8543, 2.7973) knots 0 0 0 1 2 2 2
  spline S157 degree 2 poles (-0.8543, 2.7973) (-0.8851, 2.7673) (-0.9759, 2.7308) (-1.0261, 2.7308) knots 0 0 0 1 2 2 2
  spline S158 degree 2 poles (-1.0261, 2.7308) (-1.1039, 2.7308) (-1.2141, 2.7965) (-1.2457, 2.8678) knots 0 0 0 1 2 2 2
  spline S159 degree 2 poles (-1.2457, 2.8678) (-1.2749, 2.931) (-1.2968, 3.1028) (-1.3025, 3.2025) knots 0 0 0 1 2 2 2
  line L151 (-1.3025, 3.2025) -> (-1.3268, 3.2025)
  spline S160 degree 2 poles (-1.3268, 3.2025) (-1.3705, 3.2025) (-1.4248, 3.1757) (-1.4402, 3.1514) knots 0 0 0 1 2 2 2
  spline S161 degree 2 poles (-1.4402, 3.1514) (-1.4556, 3.1271) (-1.4654, 3.0574) (-1.4654, 3.0201) knots 0 0 0 1 2 2 2
  spline S162 degree 2 poles (-1.4654, 3.0201) (-1.4654, 2.9764) (-1.4394, 2.8581) (-1.4143, 2.7989) knots 0 0 0 1 2 2 2
  line L152 (-1.4143, 2.7989) -> (-1.4143, 2.7916)
  line L153 (-1.4143, 2.7916) -> (-1.5432, 2.7916)
  spline S163 degree 2 poles (-1.5432, 2.7916) (-1.5529, 2.8265) (-1.5772, 2.9569) (-1.5772, 3.021) knots 0 0 0 1 2 2 2
  spline S164 degree 2 poles (-1.5772, 3.021) (-1.5772, 3.0987) (-1.5529, 3.2049) (-1.5213, 3.247) knots 0 0 0 1 2 2 2
  spline S165 degree 2 poles (-1.5213, 3.247) (-1.4905, 3.2884) (-1.3924, 3.3289) (-1.3219, 3.3289) knots 0 0 0 1 2 2 2
  line L154 (-1.3219, 3.3289) -> (-0.809, 3.3289)
  line L155 (-0.809, 3.3289) -> (-0.809, 3.2025)
  line L156 (-0.809, 3.2025) -> (-0.8884, 3.2025)
  line L157 (-0.9937, 3.2025) -> (-1.202, 3.2025)
  spline S166 degree 2 poles (-1.202, 3.2025) (-1.1979, 3.1571) (-1.1842, 3.0201) (-1.1712, 2.9772) knots 0 0 0 1 2 2 2
  spline S167 degree 2 poles (-1.1712, 2.9772) (-1.1558, 2.9269) (-1.0918, 2.8613) (-1.035, 2.8613) knots 0 0 0 1 2 2 2
  spline S168 degree 2 poles (-1.035, 2.8613) (-0.9702, 2.8613) (-0.9046, 2.9342) (-0.9046, 3.0039) knots 0 0 0 1 2 2 2
  spline S169 degree 2 poles (-0.9046, 3.0039) (-0.9046, 3.0631) (-0.9556, 3.1603) (-0.9937, 3.2025) knots 0 0 0 1 2 2 2
  spline S170 degree 2 poles (-0.7919, 3.8046) (-0.7919, 3.7268) (-0.8398, 3.5979) (-0.8884, 3.5517) knots 0 0 0 1 2 2 2
  spline S171 degree 2 poles (-0.8884, 3.5517) (-0.9362, 3.5056) (-1.0837, 3.4545) (-1.1825, 3.4545) knots 0 0 0 1 2 2 2
  spline S172 degree 2 poles (-1.1825, 3.4545) (-1.2814, 3.4545) (-1.4256, 3.5072) (-1.4743, 3.5517) knots 0 0 0 1 2 2 2
  spline S173 degree 2 poles (-1.4743, 3.5517) (-1.5237, 3.5963) (-1.5764, 3.7284) (-1.5764, 3.8046) knots 0 0 0 1 2 2 2
  spline S174 degree 2 poles (-1.5764, 3.8046) (-1.5764, 3.8662) (-1.5415, 3.9812) (-1.5188, 4.0258) knots 0 0 0 1 2 2 2
  line L158 (-1.5188, 4.0258) -> (-1.377, 4.0258)
  line L159 (-1.377, 4.0258) -> (-1.377, 4.0185)
  spline S175 degree 2 poles (-1.377, 4.0185) (-1.3884, 4.0047) (-1.4175, 3.9626) (-1.4329, 3.9326) knots 0 0 0 1 2 2 2
  spline S176 degree 2 poles (-1.4329, 3.9326) (-1.4459, 3.9059) (-1.4662, 3.8346) (-1.4662, 3.8022) knots 0 0 0 1 2 2 2
  spline S177 degree 2 poles (-1.4662, 3.8022) (-1.4662, 3.7041) (-1.3179, 3.585) (-1.1825, 3.585) knots 0 0 0 1 2 2 2
  spline S178 degree 2 poles (-1.1825, 3.585) (-1.0504, 3.585) (-0.9021, 3.7) (-0.9021, 3.8022) knots 0 0 0 1 2 2 2
  spline S179 degree 2 poles (-0.9021, 3.8022) (-0.9021, 3.8637) (-0.9532, 3.9756) (-0.9929, 4.0185) knots 0 0 0 1 2 2 2
  line L160 (-0.9929, 4.0185) -> (-0.9929, 4.0258)
  line L161 (-0.9929, 4.0258) -> (-0.8511, 4.0258)
  spline S180 degree 2 poles (-0.8511, 4.0258) (-0.8422, 4.0072) (-0.8171, 3.9504) (-0.8114, 3.9278) knots 0 0 0 1 2 2 2
  spline S181 degree 2 poles (-0.8114, 3.9278) (-0.8017, 3.8953) (-0.7919, 3.8443) (-0.7919, 3.8046) knots 0 0 0 1 2 2 2
  line L162 (-0.809, 4.73) -> (-0.809, 4.6036)
  line L163 (-0.809, 4.6036) -> (-1.2368, 4.6036)
  spline S182 degree 2 poles (-1.2368, 4.6036) (-1.2887, 4.6036) (-1.3778, 4.5939) (-1.4046, 4.5793) knots 0 0 0 1 2 2 2
  spline S183 degree 2 poles (-1.4046, 4.5793) (-1.4329, 4.5639) (-1.4605, 4.5088) (-1.4605, 4.4618) knots 0 0 0 1 2 2 2
  spline S184 degree 2 poles (-1.4605, 4.4618) (-1.4605, 4.4148) (-1.4103, 4.3151) (-1.3697, 4.2673) knots 0 0 0 1 2 2 2
  line L164 (-1.3697, 4.2673) -> (-0.809, 4.2673)
  line L165 (-0.809, 4.2673) -> (-0.809, 4.1409)
  line L166 (-0.809, 4.1409) -> (-1.8535, 4.1409)
  line L167 (-1.8535, 4.1409) -> (-1.8535, 4.2673)
  line L168 (-1.8535, 4.2673) -> (-1.4759, 4.2673)
  spline S185 degree 2 poles (-1.4759, 4.2673) (-1.5269, 4.324) (-1.5804, 4.4334) (-1.5804, 4.495) knots 0 0 0 1 2 2 2
  spline S186 degree 2 poles (-1.5804, 4.495) (-1.5804, 4.6052) (-1.4346, 4.73) (-1.296, 4.73) knots 0 0 0 1 2 2 2
  line L169 (-1.296, 4.73) -> (-0.809, 4.73)
  line L170 (-0.809, 5.0363) -> (-0.809, 4.9099)
  line L171 (-0.809, 4.9099) -> (-1.5594, 4.9099)
  line L172 (-1.5594, 4.9099) -> (-1.5594, 5.0363)
  line L173 (-1.5594, 5.0363) -> (-0.809, 5.0363)
  line L174 (-1.6842, 5.0453) -> (-1.6842, 4.9018)
  line L175 (-1.6842, 4.9018) -> (-1.8154, 4.9018)
  line L176 (-1.8154, 4.9018) -> (-1.8154, 5.0453)
  line L177 (-1.8154, 5.0453) -> (-1.6842, 5.0453)
  line L178 (-0.809, 5.8111) -> (-0.809, 5.6846)
  line L179 (-0.809, 5.6846) -> (-1.2368, 5.6846)
  spline S187 degree 2 poles (-1.2368, 5.6846) (-1.2887, 5.6846) (-1.3778, 5.6749) (-1.4046, 5.6603) knots 0 0 0 1 2 2 2
  spline S188 degree 2 poles (-1.4046, 5.6603) (-1.4329, 5.6449) (-1.4605, 5.5898) (-1.4605, 5.5428) knots 0 0 0 1 2 2 2
  spline S189 degree 2 poles (-1.4605, 5.5428) (-1.4605, 5.4958) (-1.4103, 5.3962) (-1.3697, 5.3483) knots 0 0 0 1 2 2 2
  line L180 (-1.3697, 5.3483) -> (-0.809, 5.3483)
  line L181 (-0.809, 5.3483) -> (-0.809, 5.2219)
  line L182 (-0.809, 5.2219) -> (-1.5594, 5.2219)
  line L183 (-1.5594, 5.2219) -> (-1.5594, 5.3483)
  line L184 (-1.5594, 5.3483) -> (-1.4759, 5.3483)
  spline S190 degree 2 poles (-1.4759, 5.3483) (-1.5269, 5.4051) (-1.5804, 5.5145) (-1.5804, 5.5761) knots 0 0 0 1 2 2 2
  spline S191 degree 2 poles (-1.5804, 5.5761) (-1.5804, 5.6863) (-1.4346, 5.8111) (-1.296, 5.8111) knots 0 0 0 1 2 2 2
  line L185 (-1.296, 5.8111) -> (-0.809, 5.8111)
  spline S192 degree 2 poles (-0.7919, 6.3143) (-0.7919, 6.1344) (-0.9937, 5.9367) (-1.1801, 5.9367) knots 0 0 0 1 2 2 2
  spline S193 degree 2 poles (-1.1801, 5.9367) (-1.3633, 5.9367) (-1.5804, 6.1287) (-1.5804, 6.2835) knots 0 0 0 1 2 2 2
  spline S194 degree 2 poles (-1.5804, 6.2835) (-1.5804, 6.3532) (-1.5399, 6.461) (-1.497, 6.5007) knots 0 0 0 1 2 2 2
  spline S195 degree 2 poles (-1.497, 6.5007) (-1.454, 6.5412) (-1.33, 6.5842) (-1.2401, 6.5842) knots 0 0 0 1 2 2 2
  line L186 (-1.2401, 6.5842) -> (-1.1712, 6.5842)
  line L187 (-1.1712, 6.5842) -> (-1.1712, 6.0647)
  spline S196 degree 2 poles (-1.1712, 6.0647) (-1.0407, 6.0647) (-0.9021, 6.196) (-0.9021, 6.3127) knots 0 0 0 1 2 2 2
  spline S197 degree 2 poles (-0.9021, 6.3127) (-0.9021, 6.354) (-0.9208, 6.4342) (-0.9354, 6.4667) knots 0 0 0 1 2 2 2
  spline S198 degree 2 poles (-0.9354, 6.4667) (-0.9516, 6.5007) (-0.9799, 6.5477) (-0.9929, 6.5631) knots 0 0 0 1 2 2 2
  line L188 (-0.9929, 6.5631) -> (-0.9929, 6.5704)
  line L189 (-0.9929, 6.5704) -> (-0.8551, 6.5704)
  spline S199 degree 2 poles (-0.8551, 6.5704) (-0.8462, 6.5485) (-0.8203, 6.4821) (-0.813, 6.4561) knots 0 0 0 1 2 2 2
  spline S200 degree 2 poles (-0.813, 6.4561) (-0.8025, 6.4197) (-0.7919, 6.3597) (-0.7919, 6.3143) knots 0 0 0 1 2 2 2
  spline S201 degree 2 poles (-1.2676, 6.461) (-1.3187, 6.4594) (-1.3932, 6.4383) (-1.4184, 6.418) knots 0 0 0 1 2 2 2
  spline S202 degree 2 poles (-1.4184, 6.418) (-1.4467, 6.3962) (-1.4767, 6.3273) (-1.4767, 6.2762) knots 0 0 0 1 2 2 2
  spline S203 degree 2 poles (-1.4767, 6.2762) (-1.4767, 6.226) (-1.4467, 6.1555) (-1.4175, 6.1263) knots 0 0 0 1 2 2 2
  spline S204 degree 2 poles (-1.4175, 6.1263) (-1.3876, 6.0979) (-1.3154, 6.0688) (-1.2676, 6.0647) knots 0 0 0 1 2 2 2
  line L190 (-1.2676, 6.0647) -> (-1.2676, 6.461)
  line L191 (-0.809, 7.2892) -> (-0.809, 7.1628)
  line L192 (-0.809, 7.1628) -> (-0.8851, 7.1628)
  spline S205 degree 2 poles (-0.8851, 7.1628) (-0.8608, 7.1336) (-0.8284, 7.0906) (-0.8146, 7.0615) knots 0 0 0 1 2 2 2
  spline S206 degree 2 poles (-0.8146, 7.0615) (-0.8017, 7.0347) (-0.7879, 6.9772) (-0.7879, 6.9391) knots 0 0 0 1 2 2 2
  spline S207 degree 2 poles (-0.7879, 6.9391) (-0.7879, 6.8775) (-0.8389, 6.7738) (-0.8884, 6.7373) knots 0 0 0 1 2 2 2
  spline S208 degree 2 poles (-0.8884, 6.7373) (-0.9378, 6.7009) (-1.0837, 6.6603) (-1.1785, 6.6603) knots 0 0 0 1 2 2 2
  spline S209 degree 2 poles (-1.1785, 6.6603) (-1.2774, 6.6603) (-1.4216, 6.7114) (-1.4759, 6.756) knots 0 0 0 1 2 2 2
  spline S210 degree 2 poles (-1.4759, 6.756) (-1.5245, 6.7973) (-1.5804, 6.9132) (-1.5804, 6.9772) knots 0 0 0 1 2 2 2
  spline S211 degree 2 poles (-1.5804, 6.9772) (-1.5804, 7.0331) (-1.5553, 7.1166) (-1.5294, 7.1628) knots 0 0 0 1 2 2 2
  line L193 (-1.5294, 7.1628) -> (-1.8535, 7.1628)
  line L194 (-1.8535, 7.1628) -> (-1.8535, 7.2892)
  line L195 (-1.8535, 7.2892) -> (-0.809, 7.2892)
  line L196 (-0.9913, 7.1628) -> (-1.4248, 7.1628)
  spline S212 degree 2 poles (-1.4248, 7.1628) (-1.4475, 7.1158) (-1.4645, 7.0412) (-1.4645, 6.9983) knots 0 0 0 1 2 2 2
  spline S213 degree 2 poles (-1.4645, 6.9983) (-1.4645, 6.901) (-1.3187, 6.7908) (-1.1809, 6.7908) knots 0 0 0 1 2 2 2
  spline S214 degree 2 poles (-1.1809, 6.7908) (-1.048, 6.7908) (-0.9078, 6.8751) (-0.9078, 6.9683) knots 0 0 0 1 2 2 2
  spline S215 degree 2 poles (-0.9078, 6.9683) (-0.9078, 7.0177) (-0.9532, 7.1182) (-0.9913, 7.1628) knots 0 0 0 1 2 2 2
  spline S216 degree 2 poles (-1.1963, 8.5307) (-1.0124, 8.5307) (-0.7879, 8.3524) (-0.7879, 8.2179) knots 0 0 0 1 2 2 2
  spline S217 degree 2 poles (-0.7879, 8.2179) (-0.7879, 8.1571) (-0.8179, 8.0704) (-0.8438, 8.0282) knots 0 0 0 1 2 2 2
  line L197 (-0.8438, 8.0282) -> (-0.809, 8.0201)
  line L198 (-0.809, 8.0201) -> (-0.809, 7.9018)
  line L199 (-0.809, 7.9018) -> (-1.8535, 7.9018)
  line L200 (-1.8535, 7.9018) -> (-1.8535, 8.0282)
  line L201 (-1.8535, 8.0282) -> (-1.4808, 8.0282)
  spline S218 degree 2 poles (-1.4808, 8.0282) (-1.5237, 8.0761) (-1.5804, 8.1871) (-1.5804, 8.2576) knots 0 0 0 1 2 2 2
  spline S219 degree 2 poles (-1.5804, 8.2576) (-1.5804, 8.3848) (-1.377, 8.5307) (-1.1963, 8.5307) knots 0 0 0 1 2 2 2
  spline S220 degree 2 poles (-1.1866, 8.4002) (-1.3211, 8.4002) (-1.4605, 8.3184) (-1.4605, 8.2276) knots 0 0 0 1 2 2 2
  spline S221 degree 2 poles (-1.4605, 8.2276) (-1.4605, 8.1765) (-1.4119, 8.0712) (-1.3746, 8.0282) knots 0 0 0 1 2 2 2
  line L202 (-1.3746, 8.0282) -> (-0.9443, 8.0282)
  spline S222 degree 2 poles (-0.9443, 8.0282) (-0.9208, 8.0761) (-0.9013, 8.1498) (-0.9013, 8.1936) knots 0 0 0 1 2 2 2
  spline S223 degree 2 poles (-0.9013, 8.1936) (-0.9013, 8.29) (-1.0383, 8.4002) (-1.1866, 8.4002) knots 0 0 0 1 2 2 2
  line L203 (-1.5594, 9.2511) -> (-0.5326, 8.8475)
  line L204 (-0.5326, 8.8475) -> (-0.5326, 8.7122)
  line L205 (-0.5326, 8.7122) -> (-0.8454, 8.8467)
  line L206 (-0.8454, 8.8467) -> (-1.5594, 8.5744)
  line L207 (-1.5594, 8.5744) -> (-1.5594, 8.7106)
  line L208 (-1.5594, 8.7106) -> (-1.0034, 8.9156)
  line L209 (-1.0034, 8.9156) -> (-1.5594, 9.1198)
  line L210 (-1.5594, 9.1198) -> (-1.5594, 9.2511)
  line L211 (-0.809, 10.512) -> (-0.809, 10.3791)
  line L212 (-0.809, 10.3791) -> (-1.2984, 10.3791)
  line L213 (-1.2984, 10.3791) -> (-1.2984, 9.9188)
  line L214 (-1.2984, 9.9188) -> (-0.809, 9.9188)
  line L215 (-0.809, 9.9188) -> (-0.809, 9.7859)
  line L216 (-0.809, 9.7859) -> (-1.809, 9.7859)
  line L217 (-1.809, 9.7859) -> (-1.809, 9.9188)
  line L218 (-1.809, 9.9188) -> (-1.4167, 9.9188)
  line L219 (-1.4167, 9.9188) -> (-1.4167, 10.3791)
  line L220 (-1.4167, 10.3791) -> (-1.809, 10.3791)
  line L221 (-1.809, 10.3791) -> (-1.809, 10.512)
  line L222 (-1.809, 10.512) -> (-0.809, 10.512)
  spline S224 degree 2 poles (-1.1842, 11.3216) (-0.9945, 11.3216) (-0.7879, 11.1393) (-0.7879, 10.9869) knots 0 0 0 1 2 2 2
  spline S225 degree 2 poles (-0.7879, 10.9869) (-0.7879, 10.8305) (-1.001, 10.6514) (-1.1842, 10.6514) knots 0 0 0 1 2 2 2
  spline S226 degree 2 poles (-1.1842, 10.6514) (-1.3722, 10.6514) (-1.5804, 10.8362) (-1.5804, 10.9869) knots 0 0 0 1 2 2 2
  spline S227 degree 2 poles (-1.5804, 10.9869) (-1.5804, 11.1393) (-1.373, 11.3216) (-1.1842, 11.3216) knots 0 0 0 1 2 2 2
  spline S228 degree 2 poles (-1.1842, 11.1911) (-1.33, 11.1911) (-1.4718, 11.085) (-1.4718, 10.9869) knots 0 0 0 1 2 2 2
  spline S229 degree 2 poles (-1.4718, 10.9869) (-1.4718, 10.8889) (-1.33, 10.7819) (-1.1842, 10.7819) knots 0 0 0 1 2 2 2
  spline S230 degree 2 poles (-1.1842, 10.7819) (-1.0423, 10.7819) (-0.8965, 10.8889) (-0.8965, 10.9869) knots 0 0 0 1 2 2 2
  spline S231 degree 2 poles (-0.8965, 10.9869) (-0.8965, 11.0842) (-1.0399, 11.1911) (-1.1842, 11.1911) knots 0 0 0 1 2 2 2
  line L223 (-0.809, 12.0347) -> (-0.809, 11.9083)
  line L224 (-0.809, 11.9083) -> (-0.8916, 11.9083)
  spline S232 degree 2 poles (-0.8916, 11.9083) (-0.8406, 11.85) (-0.7879, 11.7454) (-0.7879, 11.6806) knots 0 0 0 1 2 2 2
  spline S233 degree 2 poles (-0.7879, 11.6806) (-0.7879, 11.632) (-0.8203, 11.5453) (-0.8551, 11.5137) knots 0 0 0 1 2 2 2
  spline S234 degree 2 poles (-0.8551, 11.5137) (-0.89, 11.4812) (-0.9962, 11.4456) (-1.0723, 11.4456) knots 0 0 0 1 2 2 2
  line L225 (-1.0723, 11.4456) -> (-1.5594, 11.4456)
  line L226 (-1.5594, 11.4456) -> (-1.5594, 11.572)
  line L227 (-1.5594, 11.572) -> (-1.1315, 11.572)
  spline S235 degree 2 poles (-1.1315, 11.572) (-1.0715, 11.572) (-0.9929, 11.5809) (-0.9637, 11.5963) knots 0 0 0 1 2 2 2
  spline S236 degree 2 poles (-0.9637, 11.5963) (-0.9346, 11.6117) (-0.9078, 11.6644) (-0.9078, 11.7138) knots 0 0 0 1 2 2 2
  spline S237 degree 2 poles (-0.9078, 11.7138) (-0.9078, 11.76) (-0.9605, 11.8645) (-0.9986, 11.9083) knots 0 0 0 1 2 2 2
  line L228 (-0.9986, 11.9083) -> (-1.5594, 11.9083)
  line L229 (-1.5594, 11.9083) -> (-1.5594, 12.0347)
  line L230 (-1.5594, 12.0347) -> (-0.809, 12.0347)
  line L231 (-0.809, 12.7949) -> (-0.809, 12.6684)
  line L232 (-0.809, 12.6684) -> (-0.8851, 12.6684)
  spline S238 degree 2 poles (-0.8851, 12.6684) (-0.8608, 12.6393) (-0.8284, 12.5963) (-0.8146, 12.5671) knots 0 0 0 1 2 2 2
  spline S239 degree 2 poles (-0.8146, 12.5671) (-0.8017, 12.5404) (-0.7879, 12.4829) (-0.7879, 12.4448) knots 0 0 0 1 2 2 2
  spline S240 degree 2 poles (-0.7879, 12.4448) (-0.7879, 12.3832) (-0.8389, 12.2795) (-0.8884, 12.243) knots 0 0 0 1 2 2 2
  spline S241 degree 2 poles (-0.8884, 12.243) (-0.9378, 12.2065) (-1.0837, 12.166) (-1.1785, 12.166) knots 0 0 0 1 2 2 2
  spline S242 degree 2 poles (-1.1785, 12.166) (-1.2774, 12.166) (-1.4216, 12.2171) (-1.4759, 12.2616) knots 0 0 0 1 2 2 2
  spline S243 degree 2 poles (-1.4759, 12.2616) (-1.5245, 12.303) (-1.5804, 12.4188) (-1.5804, 12.4829) knots 0 0 0 1 2 2 2
  spline S244 degree 2 poles (-1.5804, 12.4829) (-1.5804, 12.5388) (-1.5553, 12.6222) (-1.5294, 12.6684) knots 0 0 0 1 2 2 2
  line L233 (-1.5294, 12.6684) -> (-1.8535, 12.6684)
  line L234 (-1.8535, 12.6684) -> (-1.8535, 12.7949)
  line L235 (-1.8535, 12.7949) -> (-0.809, 12.7949)
  line L236 (-0.9913, 12.6684) -> (-1.4248, 12.6684)
  spline S245 degree 2 poles (-1.4248, 12.6684) (-1.4475, 12.6214) (-1.4645, 12.5469) (-1.4645, 12.5039) knots 0 0 0 1 2 2 2
  spline S246 degree 2 poles (-1.4645, 12.5039) (-1.4645, 12.4067) (-1.3187, 12.2965) (-1.1809, 12.2965) knots 0 0 0 1 2 2 2
  spline S247 degree 2 poles (-1.1809, 12.2965) (-1.048, 12.2965) (-0.9078, 12.3808) (-0.9078, 12.4739) knots 0 0 0 1 2 2 2
  spline S248 degree 2 poles (-0.9078, 12.4739) (-0.9078, 12.5234) (-0.9532, 12.6239) (-0.9913, 12.6684) knots 0 0 0 1 2 2 2
  spline S249 degree 2 poles (-0.7919, 13.3038) (-0.7919, 13.1239) (-0.9937, 12.9261) (-1.1801, 12.9261) knots 0 0 0 1 2 2 2
  spline S250 degree 2 poles (-1.1801, 12.9261) (-1.3633, 12.9261) (-1.5804, 13.1182) (-1.5804, 13.273) knots 0 0 0 1 2 2 2
  spline S251 degree 2 poles (-1.5804, 13.273) (-1.5804, 13.3427) (-1.5399, 13.4504) (-1.497, 13.4902) knots 0 0 0 1 2 2 2
  spline S252 degree 2 poles (-1.497, 13.4902) (-1.454, 13.5307) (-1.33, 13.5736) (-1.2401, 13.5736) knots 0 0 0 1 2 2 2
  line L237 (-1.2401, 13.5736) -> (-1.1712, 13.5736)
  line L238 (-1.1712, 13.5736) -> (-1.1712, 13.0542)
  spline S253 degree 2 poles (-1.1712, 13.0542) (-1.0407, 13.0542) (-0.9021, 13.1855) (-0.9021, 13.3022) knots 0 0 0 1 2 2 2
  spline S254 degree 2 poles (-0.9021, 13.3022) (-0.9021, 13.3435) (-0.9208, 13.4237) (-0.9354, 13.4561) knots 0 0 0 1 2 2 2
  spline S255 degree 2 poles (-0.9354, 13.4561) (-0.9516, 13.4902) (-0.9799, 13.5372) (-0.9929, 13.5526) knots 0 0 0 1 2 2 2
  line L239 (-0.9929, 13.5526) -> (-0.9929, 13.5598)
  line L240 (-0.9929, 13.5598) -> (-0.8551, 13.5598)
  spline S256 degree 2 poles (-0.8551, 13.5598) (-0.8462, 13.538) (-0.8203, 13.4715) (-0.813, 13.4456) knots 0 0 0 1 2 2 2
  spline S257 degree 2 poles (-0.813, 13.4456) (-0.8025, 13.4091) (-0.7919, 13.3492) (-0.7919, 13.3038) knots 0 0 0 1 2 2 2
  spline S258 degree 2 poles (-1.2676, 13.4504) (-1.3187, 13.4488) (-1.3932, 13.4278) (-1.4184, 13.4075) knots 0 0 0 1 2 2 2
  spline S259 degree 2 poles (-1.4184, 13.4075) (-1.4467, 13.3856) (-1.4767, 13.3167) (-1.4767, 13.2657) knots 0 0 0 1 2 2 2
  spline S260 degree 2 poles (-1.4767, 13.2657) (-1.4767, 13.2154) (-1.4467, 13.1449) (-1.4175, 13.1158) knots 0 0 0 1 2 2 2
  spline S261 degree 2 poles (-1.4175, 13.1158) (-1.3876, 13.0874) (-1.3154, 13.0582) (-1.2676, 13.0542) knots 0 0 0 1 2 2 2
  line L241 (-1.2676, 13.0542) -> (-1.2676, 13.4504)
  line L242 (-0.809, 14.3232) -> (-0.809, 14.1571)
  line L243 (-0.809, 14.1571) -> (-1.1712, 13.8783)
  line L244 (-1.1712, 13.8783) -> (-1.1226, 13.8281)
  line L245 (-1.1226, 13.8281) -> (-0.809, 13.8281)
  line L246 (-0.809, 13.8281) -> (-0.809, 13.7017)
  line L247 (-0.809, 13.7017) -> (-1.8535, 13.7017)
  line L248 (-1.8535, 13.7017) -> (-1.8535, 13.8281)
  line L249 (-1.8535, 13.8281) -> (-1.2425, 13.8281)
  line L250 (-1.2425, 13.8281) -> (-1.5594, 14.1247)
  line L251 (-1.5594, 14.1247) -> (-1.5594, 14.2819)
  line L252 (-1.5594, 14.2819) -> (-1.2457, 13.9739)
  line L253 (-1.2457, 13.9739) -> (-0.809, 14.3232)
  point P0 (0, 0)
  dimension "d33" = 15
  dimension "d34" = 3.5
  dimension "d35" = 0.5
  constraints: 1 point on line, 1 vertical alignment, 2 other
  measures "d33" distance of L14.start L14.end
  measures "d34" distance of L16.end L14.start
  measures "d35" distance from line of A0.centre L17